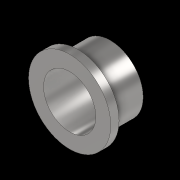
# Autodesk Inventor part: brushing
Saved by Autodesk Inventor 2022.2 (Build 262287010, 287A)
## iProperties
Created: 2022-04-27
Part Number: brushing
Material: Stainless Steel
Document SubType Name: Modeling
Designer: Árni Þór Þorgeirsson
Density: 8 g/cm^3
Appearance: Semi-Polished
Author: Árni Þór Þorgeirsson
Autodesk Inventor part; units mm, degrees
ref_plane "YZ Plane" through (0, 0, 0) normal (1, 0, 0) x (0, 1, 0)
ref_plane "XZ Plane" through (0, 0, 0) normal (0, 1, 0) x (-1, 0, 0)
ref_plane "XY Plane" through (0, 0, 0) normal (0, 0, 1) x (1, 0, 0)
sketch "Sketch1" plane through (0, 0, 0) normal (0, 0, 1) x (1, 0, 0)
  circle A0 centre (0, 0) radius 3.95
  circle A1 centre (0, 0) radius 3.15
  dimension "d0" = 7.9
  dimension "d1" = 6.3
  constraints: 2 centre point, 2 coincident
  measures "d0" diameter of A0
  measures "d1" diameter of A1
extrude "Extrusion1" add sketch "Sketch1" along normal blind 4.9
sketch "Sketch2" plane through (0, 0, 4.9) normal (0, 0, 1) x (1, 0, 0)
  circle A0 centre (0, 0) radius 4.95
  circle A1 centre (0, 0) radius 3.15 projected
  dimension "d4" = 9.9
  constraints: 1 centre point, 1 coincident
  measures "d4" diameter of A0
extrude "Extrusion2" add sketch "Sketch2" against normal blind 1
body "Solid1"
